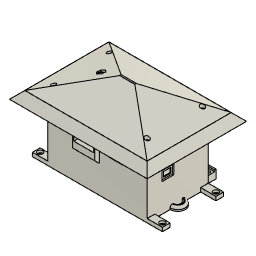
Smart Garden Enclosure v9 (Autodesk Fusion 360 design; units mm, degrees)
Autodesk Fusion 360 part; units mm, degrees
note: some values were not read from the file. Set by a fixed rule: which face or edge a step refers to.
(part 1 of 2)
sketch "Sketch1" plane through (0, 0, 0) normal (0, 0, 1) x (1, 0, 0)
  line L0 (0, 0) -> (130, 0)
  line L1 (130, 0) -> (130, 80)
  line L2 (130, 80) -> (0, 80)
  line L3 (0, 80) -> (0, 0)
  dimension "d1" = 130
  dimension "d2" = 80
  constraint horizontal L0
  constraint vertical L1
  constraint horizontal L2
  constraint vertical L3
  constraint coincident L0.start L3.end
  measures "d1" distance of L0.start L0.end
  measures "d2" distance of L0.start L2.end
extrude "Extrude1" add sketch "Sketch1" along normal blind 60 makes body 1
shell "Shell1" thickness 2 removed faces 1 at (43.3333, 26.6667, 60) on bodies 1
extrude "Extrude2" add 1 faces at (44, 52.6667, 2) along direction (0, 0, 1) blind 8 on bodies 1 bodies 1
sketch "Sketch2" plane through (0, 0, 0) normal (0, -1, 0) x (1, 0, 0)
  line L0 (0, 0) -> (130, 0)
  line L1 (130, 0) -> (130, 60)
  line L2 (130, 60) -> (0, 60)
  line L3 (0, 60) -> (0, 0)
  line L4 (2, 10) -> (128, 10)
  line L5 (128, 10) -> (2, 10)
  line L6 (4.76, 10) -> (125.26, 10)
  line L7 (4.76, 10) -> (4.76, 13.5)
  line L8 (4.76, 13.5) -> (125.26, 13.5)
  line L9 (125.26, 13.5) -> (125.26, 10)
  line L10 (16.01, 13.5) -> (33.01, 13.5)
  line L11 (33.01, 13.5) -> (33.01, 25)
  line L12 (33.01, 25) -> (16.01, 25)
  line L13 (16.01, 25) -> (16.01, 13.5)
  line L14 (43.01, 13.5) -> (60.01, 13.5)
  line L15 (60.01, 13.5) -> (60.01, 25)
  line L16 (60.01, 25) -> (43.01, 25)
  line L17 (43.01, 25) -> (43.01, 13.5)
  line L18 (70.01, 13.5) -> (87.01, 13.5)
  line L19 (87.01, 13.5) -> (87.01, 25)
  line L20 (87.01, 25) -> (70.01, 25)
  line L21 (70.01, 25) -> (70.01, 13.5)
  line L22 (97.01, 13.5) -> (114.01, 13.5)
  line L23 (114.01, 13.5) -> (114.01, 25)
  line L24 (114.01, 25) -> (97.01, 25)
  line L25 (97.01, 25) -> (97.01, 13.5)
  dimension "d27" = 120.5
  dimension "d29" = 3.5
  dimension "d30" = 17
  dimension "d31" = 11.5
  dimension "d32" = 17
  dimension "d33" = 11.5
  dimension "d35" = 17
  dimension "d36" = 11.5
  dimension "d37" = 17
  dimension "d38" = 11.5
  dimension "d42" = 11.25
  dimension "d43" = 11.25
  dimension "d44" = 10
  dimension "d45" = 10
  constraint coincident L4 L6.start
  constraint parallel L5 L6
  constraint perpendicular L5 L7
  constraint perpendicular L7 L8
  constraint perpendicular L8 L9
  constraint horizontal L10
  constraint vertical L11
  constraint horizontal L12
  constraint vertical L13
  constraint coincident L8 L10.start
  constraint horizontal L14
  constraint vertical L15
  constraint horizontal L16
  constraint vertical L17
  constraint coincident L8 L14.start
  constraint horizontal L18
  constraint vertical L19
  constraint horizontal L20
  constraint vertical L21
  constraint coincident L8 L18.start
  constraint horizontal L22
  constraint vertical L23
  constraint horizontal L24
  constraint vertical L25
  constraint coincident L8 L22.start
  measures "d27" distance of L6.start L6.end
  measures "d29" distance of L6.start L7.end
  measures "d30" distance of L10.start L10.end
  measures "d31" distance of L10.start L12.end
  measures "d32" distance of L14.start L14.end
  measures "d33" distance of L14.start L16.end
  measures "d35" distance of L18.start L18.end
  measures "d36" distance of L18.start L20.end
  measures "d37" distance of L22.start L22.end
  measures "d38" distance of L22.start L24.end
  measures "d42" distance of L9 L23
  measures "d43" distance of L7 L13
  measures "d44" distance of L11 L17
  measures "d45" distance of L15 L21
extrude "Extrude4" cut sketch "Sketch2" against normal blind 95 contours L4 L5 L6 L7 L8 L9 L10 L14 L18 L22 | L8 L10 L11 L12 L13 | L8 L22 L23 L24 L25 | L8 L14 L15 L16 L17 | L8 L18 L19 L20 L21 bodies 1
sketch "Sketch3" plane through (0, 0, 0) normal (0, -1, 0) x (1, 0, 0)
  line L0 (97.01, 25) -> (114.01, 25)
  line L1 (114.01, 25) -> (114.01, 13.5)
  line L2 (114.01, 13.5) -> (125.26, 13.5)
  line L3 (125.26, 13.5) -> (125.26, 10)
  line L4 (125.26, 10) -> (4.76, 10)
  line L5 (4.76, 10) -> (4.76, 13.5)
  line L6 (4.76, 13.5) -> (16.01, 13.5)
  line L7 (16.01, 13.5) -> (16.01, 25)
  line L8 (16.01, 25) -> (33.01, 25)
  line L9 (33.01, 25) -> (33.01, 13.5)
  line L10 (33.01, 13.5) -> (43.01, 13.5)
  line L11 (43.01, 13.5) -> (43.01, 25)
  line L12 (43.01, 25) -> (60.01, 25)
  line L13 (60.01, 25) -> (60.01, 13.5)
  line L14 (60.01, 13.5) -> (70.01, 13.5)
  line L15 (70.01, 13.5) -> (70.01, 25)
  line L16 (70.01, 25) -> (87.01, 25)
  line L17 (87.01, 25) -> (87.01, 13.5)
  line L18 (87.01, 13.5) -> (97.01, 13.5)
  line L19 (97.01, 13.5) -> (97.01, 25)
  line L20 (0, 0) -> (130, 0)
  line L21 (130, 0) -> (130, 60)
  line L22 (130, 60) -> (0, 60)
  line L23 (0, 60) -> (0, 0)
  line L24 (4.76, 10) -> (125.26, 10)
  line L25 (125.26, 10) -> (125.26, 0)
  line L26 (4.76, 10) -> (4.76, 0)
  constraint coincident L4.end L5.start
  constraint coincident L3.end L4.start
  constraint coincident L20 L25.end
  constraint perpendicular L20 L25
  constraint coincident L20 L26.end
  constraint perpendicular L20 L26
extrude "Extrude5" add sketch "Sketch3" against normal blind 93 contours L4 L20 L24 L25 L26 bodies 1
sketch "Sketch4" plane through (0, 0, 10) normal (0, 0, 1) x (-1, 0, 0)
  line L0 (-125.26, -2) -> (-128, -2)
  line L1 (-128, -2) -> (-128, -78)
  line L2 (-128, -78) -> (-125.26, -78)
  line L3 (-2, -78) -> (-2, -2)
  line L4 (-2, -2) -> (-4.76, -2)
  line L5 (-4.76, -2) -> (-4.76, 0)
  line L6 (-4.76, -93) -> (-4.76, -80)
  line L7 (-125.26, -80) -> (-125.26, -93)
  line L8 (-125.26, 0) -> (-125.26, -2)
  circle A0 centre (-9.51, 7.0656) radius 2
  circle A1 centre (-120.51, 6.9823) radius 2
  line L9 (-125.26, -93) -> (-4.76, -93)
  line L10 (-4.76, -78) -> (-2, -78)
  line L11 (-4.76, 0) -> (-125.26, 0)
  line L12 (-125.26, -78) -> (-125.26, -80)
  line L13 (-4.76, -80) -> (-4.76, -78)
  dimension "d51" = 4
  dimension "d52" = 4
  dimension "d53" = 111
  dimension "d54" = 4.75
  measures "d51" diameter of A0
  measures "d52" diameter of A1
  measures "d53" horizontal distance of A0.centre A1.centre
  measures "d54" distance of L6 A0.centre
extrude "Extrude6" cut sketch "Sketch4" against normal blind 6 contours A0 | A1 bodies 1
sketch "Sketch5" plane through (0, 0, 10) normal (0, 0, 1) x (-1, 0, 0)
  line L0 (-125.26, -2) -> (-128, -2)
  line L1 (-128, -2) -> (-128, -78)
  line L2 (-128, -78) -> (-125.26, -78)
  line L3 (-2, -78) -> (-2, -2)
  line L4 (-2, -2) -> (-4.76, -2)
  line L5 (-4.76, -2) -> (-4.76, 0)
  line L6 (-4.76, -93) -> (-4.76, -80)
  line L7 (-125.26, -80) -> (-125.26, -93)
  line L8 (-125.26, 0) -> (-125.26, -2)
  line L9 (-9.51, 7.0656) -> (-9.51, -78)
  line L10 (-120.51, 6.9823) -> (-120.51, -78)
  circle A0 centre (-9.51, -44.9344) radius 2
  circle A1 centre (-120.51, -45.0177) radius 2
  line L11 (-125.26, -93) -> (-4.76, -93)
  line L12 (-4.76, -78) -> (-2, -78)
  line L13 (-4.76, 0) -> (-125.26, 0)
  line L14 (-125.26, -78) -> (-125.26, -80)
  line L15 (-4.76, -80) -> (-4.76, -78)
  dimension "d57" = 4
  dimension "d58" = 4
  dimension "d59" = 52
  dimension "d60" = 52
  constraint coincident L2 L9.end
  constraint perpendicular L2 L9
  constraint coincident L2 L10.end
  constraint perpendicular L2 L10
  constraint coincident L9 A0.centre
  constraint coincident L10 A1.centre
  measures "d57" diameter of A0
  measures "d58" diameter of A1
  measures "d59" distance of L9.start A0.centre
  measures "d60" distance of L10.start A1.centre
extrude "Extrude7" cut sketch "Sketch5" against normal blind 5 contours L9 A0 | L9 A0 | L10 A1 | L10 A1 bodies 1
ref_plane "WorkPlane1" through (65, 46.5, 28) normal (0, 0, 1) x (1, 0, 0)
sketch "Sketch6" plane through (65, 32.5, 28) normal (0, 0, 1) x (1, 0, 0)
  line L0 (-63, 45.5) -> (63, 45.5)
  line L1 (63, 45.5) -> (63, -30.5)
  line L2 (63, -30.5) -> (-63, -30.5)
  line L3 (-63, -30.5) -> (-63, 45.5)
  line L4 (-65, 47.5) -> (-65, -32.5)
  line L5 (-65, -32.5) -> (65, -32.5)
  line L6 (65, -32.5) -> (65, 47.5)
  line L7 (65, 47.5) -> (-65, 47.5)
  line L8 (-63, -30.5) -> (-63, 45.5)
  line L9 (-63, -30.5) -> (-53, -30.5)
  line L10 (-53, -30.5) -> (-53, 45.5)
  line L11 (-53, 45.5) -> (-63, 45.5)
  line L12 (-53, -30.5) -> (-53, -18.5)
  line L13 (-53, -18.5) -> (-63, -18.5)
  line L14 (-53, 45.5) -> (-53, 30)
  line L15 (-53, 45.5) -> (-53, 33.5)
  line L16 (-53, 33.5) -> (-63, 33.5)
  line L17 (63, -30.5) -> (53, -30.5)
  line L18 (53, -30.5) -> (53, -18.5)
  line L19 (53, -18.5) -> (63, -18.5)
  line L20 (53, 45.5) -> (63, 45.5)
  line L21 (53, 45.5) -> (53, 33.5)
  line L22 (53, 33.5) -> (63, 33.5)
  line L23 (-53, -18.5) -> (-40, -18.5)
  line L24 (-40, -18.5) -> (-40, -30.5)
  line L25 (53, -18.5) -> (40, -18.5)
  line L26 (40, -18.5) -> (40, -30.5)
  line L27 (-53, 33.5) -> (-40, 33.5)
  line L28 (-40, 33.5) -> (-40, 45.5)
  line L29 (53, 33.5) -> (40, 33.5)
  line L30 (40, 33.5) -> (40, 45.5)
  dimension "d64" = 10
  dimension "d67" = 12
  dimension "d68" = 10
  dimension "d69" = 12
  dimension "d283" = 12
  dimension "d284" = 12
  constraint coincident L2.end L3.start
  constraint coincident L0.start L3.end
  constraint coincident L2 L9.end
  constraint perpendicular L3 L9
  constraint coincident L0 L10.end
  constraint perpendicular L0 L10
  constraint coincident L10 L12.end
  constraint perpendicular L9 L12
  constraint coincident L8 L13.end
  constraint perpendicular L8 L13
  constraint coincident L10 L14.end
  constraint perpendicular L11 L14
  constraint perpendicular L11 L15
  constraint coincident L8 L16.end
  constraint perpendicular L8 L16
  constraint coincident L1.end L2.start
  constraint coincident L2 L17.end
  constraint perpendicular L2 L18
  constraint coincident L1 L19.end
  constraint perpendicular L1 L19
  constraint coincident L0 L20.start
  constraint coincident L0.end L1.start
  constraint perpendicular L1 L20
  constraint perpendicular L20 L21
  constraint coincident L1 L22.end
  constraint perpendicular L1 L22
  constraint perpendicular L10 L23
  constraint coincident L2 L24.end
  constraint perpendicular L2 L24
  constraint perpendicular L18 L25
  constraint coincident L2 L26.end
  constraint perpendicular L2 L26
  constraint perpendicular L14 L27
  constraint coincident L0 L28.end
  constraint perpendicular L0 L28
  constraint perpendicular L21 L29
  constraint coincident L0 L30.end
  constraint perpendicular L0 L30
  measures "d64" distance of L8 L10
  measures "d67" distance of L10.end L15.end
  measures "d68" distance of L1.end L17.end
  measures "d69" distance of L20.start L21.end
  measures "d283" distance of L17 L19
  measures "d284" distance of L9 L13
extrude "Extrude8" add sketch "Sketch6" along normal blind 5 and the other way blind 7 contours L0 L3 L8 L10 L11 L14 L15 L16 | L2 L3 L8 L9 L10 L12 L13 | L0 L1 L20 L21 L22 | L1 L2 L17 L18 L19 bodies 1
sketch "Sketch7" plane through (0, 0, 33) normal (0, 0, 1) x (-1, 0, 0)
  line L0 (-2, -2) -> (-12, -2)
  line L1 (-12, -14) -> (-2, -14)
  line L2 (-2, -14) -> (-2, -2)
  line L3 (-12, -78) -> (-2, -78)
  line L4 (-2, -78) -> (-2, -66)
  line L5 (-2, -66) -> (-12, -66)
  line L6 (-118, -66) -> (-128, -66)
  line L7 (-128, -66) -> (-128, -78)
  line L8 (-128, -78) -> (-118, -78)
  line L9 (-118, -2) -> (-128, -2)
  line L10 (-128, -2) -> (-128, -14)
  line L11 (-128, -14) -> (-118, -14)
  line L12 (-2, -2) -> (-128, -2)
  line L13 (-128, -2) -> (-128, -78)
  line L14 (-128, -78) -> (-2, -78)
  line L15 (-2, -78) -> (-2, -2)
  line L16 (-3, -77) -> (-3, -3)
  line L17 (-3, -3) -> (-127, -3)
  line L18 (-127, -3) -> (-127, -77)
  line L19 (-127, -77) -> (-3, -77)
  line L20 (-12, -2) -> (-12, -14)
  line L21 (-12, -66) -> (-12, -78)
  line L22 (-118, -78) -> (-118, -66)
  line L23 (-118, -14) -> (-118, -2)
  dimension "d71" = -1
  constraint horizontal L12
  constraint vertical L13
  constraint horizontal L14
  constraint vertical L15
  constraint coincident L7.end L8.start
  constraint coincident L0.start L2.end
extrude "Extrude9" add sketch "Sketch7" along normal blind 7 separate body contours L1 L5 L6 L11 L16 L17 L18 L19 L20 L21 L22 L23 | L1 L16 L17 L20 | L11 L17 L18 L23 | L5 L16 L19 L21 | L6 L18 L19 L22 makes body 2
sketch "Sketch8" plane through (0, 0, 40) normal (0, 0, 1) x (-1, 0, 0)
  line L0 (-127, -77) -> (-3, -77)
  line L1 (-3, -77) -> (-3, -3)
  line L2 (-3, -3) -> (-127, -3)
  line L3 (-127, -3) -> (-127, -77)
  line L4 (-12, -78) -> (-2, -78)
  line L5 (-2, -78) -> (-2, -66)
  line L6 (-2, -66) -> (-12, -66)
  line L7 (-2, -2) -> (-12, -2)
  line L8 (-12, -14) -> (-2, -14)
  line L9 (-2, -14) -> (-2, -2)
  line L10 (-118, -66) -> (-128, -66)
  line L11 (-128, -66) -> (-128, -78)
  line L12 (-128, -78) -> (-118, -78)
  line L13 (-118, -2) -> (-128, -2)
  line L14 (-128, -2) -> (-128, -14)
  line L15 (-128, -14) -> (-118, -14)
  circle A0 centre (-7, -71.7119) radius 1.5
  circle A1 centre (-6.9931, -7.787) radius 1.5
  circle A2 centre (-123.226, -7.2087) radius 1.5
  line L16 (-12, -66) -> (-12, -78)
  line L17 (-12, -2) -> (-12, -14)
  line L18 (-118, -78) -> (-118, -66)
  line L19 (-118, -14) -> (-118, -2)
  dimension "d74" = 3
  dimension "d75" = 3
  dimension "d77" = 3
  measures "d74" diameter of A0
  measures "d75" diameter of A1
  measures "d77" diameter of A2
sketch "Sketch9" plane through (0, 80, 0) normal (0, 1, 0) x (-1, 0, 0)
  line L0 (-4.76, 0) -> (0, 0)
  line L1 (0, 0) -> (0, 60)
  line L2 (0, 60) -> (-130, 60)
  line L3 (-130, 60) -> (-130, 0)
  line L4 (-127, 40) -> (-3, 40)
  line L5 (-3, 40) -> (-127, 40)
  line L6 (-114.01, 25) -> (-97.01, 25)
  line L7 (-97.01, 25) -> (-97.01, 13.5)
  line L8 (-97.01, 13.5) -> (-87.01, 13.5)
  line L9 (-87.01, 13.5) -> (-87.01, 25)
  line L10 (-87.01, 25) -> (-70.01, 25)
  line L11 (-70.01, 25) -> (-70.01, 13.5)
  line L12 (-70.01, 13.5) -> (-60.01, 13.5)
  line L13 (-60.01, 13.5) -> (-60.01, 25)
  line L14 (-60.01, 25) -> (-43.01, 25)
  line L15 (-43.01, 25) -> (-43.01, 13.5)
  line L16 (-43.01, 13.5) -> (-33.01, 13.5)
  line L17 (-33.01, 13.5) -> (-33.01, 25)
  line L18 (-33.01, 25) -> (-16.01, 25)
  line L19 (-16.01, 25) -> (-16.01, 13.5)
  line L20 (-16.01, 13.5) -> (-4.76, 13.5)
  line L21 (-4.76, 13.5) -> (-4.76, 10)
  line L22 (-125.26, 10) -> (-125.26, 13.5)
  line L23 (-125.26, 13.5) -> (-114.01, 13.5)
  line L24 (-114.01, 13.5) -> (-114.01, 25)
  line L25 (-4.76, 10) -> (-4.76, 0)
  line L26 (-130, 0) -> (-125.26, 0)
  line L27 (-125.26, 0) -> (-125.26, 10)
sketch "Sketch10" plane through (0, 0, 40) normal (0, 0, 1) x (-1, 0, 0)
  line L0 (-127, -77) -> (-3, -77)
  line L1 (-3, -77) -> (-3, -3)
  line L2 (-3, -3) -> (-127, -3)
  line L3 (-127, -3) -> (-127, -77)
  circle A0 centre (-7, -71.7119) radius 3.5
  circle A1 centre (-6.9931, -7.787) radius 3.5
  circle A2 centre (-123.226, -7.2087) radius 3.5
  dimension "d80" = 7
  dimension "d81" = 7
  dimension "d83" = 7
  measures "d80" diameter of A0
  measures "d81" diameter of A1
  measures "d83" diameter of A2
sketch "Sketch14" plane through (0, 0, 40) normal (0, 0, 1) x (-1, 0, 0)
  line L0 (-127, -77) -> (-3, -77)
  line L1 (-3, -77) -> (-3, -3)
  line L2 (-3, -3) -> (-127, -3)
  line L3 (-127, -3) -> (-127, -77)
  line L4 (-127, -77) -> (-30, -77)
  line L5 (-30, -77) -> (-30, -13)
  line L6 (-30, -13) -> (-127, -13)
  line L7 (-127, -13) -> (-127, -77)
  dimension "d101" = 97
  dimension "d102" = 64
  constraint horizontal L4
  constraint vertical L5
  constraint horizontal L6
  constraint vertical L7
  constraint coincident L0.start L3.end
  measures "d101" distance of L0.start L4.end
  measures "d102" distance of L0.start L6.end
extrude "Extrude15" cut sketch "Sketch14" against normal blind 2 contours L0 L3 L4 L5 L6 L7 bodies 2
sketch "Sketch15" plane through (128, 0, 0) normal (-1, 0, 0) x (0, -1, 0)
  line L0 (-78, 33) -> (-66, 33)
  line L1 (-66, 33) -> (-66, 21)
  line L2 (-78, 21) -> (-78, 10)
  line L3 (-78, 10) -> (-2, 10)
  line L4 (-2, 10) -> (-2, 21)
  line L5 (-14, 21) -> (-14, 33)
  line L6 (-14, 33) -> (-2, 33)
  line L7 (-2, 33) -> (-2, 60)
  line L8 (-2, 60) -> (-78, 60)
  line L9 (-78, 60) -> (-78, 33)
  line L10 (-32, 40) -> (-22.5, 40)
  line L11 (-22.5, 40) -> (-22.5, 46.5)
  line L12 (-22.5, 46.5) -> (-32, 46.5)
  line L13 (-32, 46.5) -> (-32, 40)
  line L14 (-66, 21) -> (-78, 21)
  line L15 (-2, 21) -> (-14, 21)
  point P0 (-77, 38)
  point P1 (-13, 38)
  dimension "d105" = 9.5
  dimension "d106" = 6.5
  constraint horizontal L10
  constraint vertical L11
  constraint horizontal L12
  constraint vertical L13
  measures "d105" distance of L10.start L10.end
  measures "d106" distance of L10.start L12.end
extrude "Extrude16" cut sketch "Sketch15" against normal blind 2 contours L10 L11 L12 L13 bodies 1
sketch "Sketch16" plane through (130, 0, 0) normal (1, 0, 0) x (0, 1, 0)
  line L0 (32, 40) -> (22.5, 40)
  line L1 (22.5, 40) -> (22.5, 46.5)
  line L2 (22.5, 46.5) -> (32, 46.5)
  line L3 (32, 46.5) -> (32, 40)
  line L4 (0, 0) -> (80, 0)
  line L5 (80, 0) -> (80, 60)
  line L6 (80, 60) -> (0, 60)
  line L7 (0, 60) -> (0, 0)
  line L8 (34, 38) -> (20.5, 38)
  line L9 (20.5, 38) -> (20.5, 48.5)
  line L10 (20.5, 48.5) -> (34, 48.5)
  line L11 (34, 48.5) -> (34, 38)
  dimension "d110" = -2
extrude "Extrude17" cut sketch "Sketch16" against normal blind 1 contours L8 L9 L10 L11 bodies 1
chamfer "Chamfer4" distance 1 angle 45 4 edges at (130, 27.25, 48.5) (130, 34, 43.25) (130, 20.5, 43.25) (130, 27.25, 38) on bodies 1
sketch "Sketch17" plane through (0, 80, 0) normal (0, 1, 0) x (-1, 0, 0)
  line L0 (-117, 41) -> (-101.5, 41)
  line L1 (-101.5, 41) -> (-101.5, 49)
  line L2 (-101.5, 49) -> (-117, 49)
  line L3 (-117, 49) -> (-117, 41)
  line L4 (-96.5, 41) -> (-81, 41)
  line L5 (-81, 41) -> (-81, 49)
  line L6 (-81, 49) -> (-96.5, 49)
  line L7 (-96.5, 49) -> (-96.5, 41)
  line L8 (-76, 41) -> (-60.5, 41)
  line L9 (-60.5, 41) -> (-60.5, 49)
  line L10 (-60.5, 49) -> (-76, 49)
  line L11 (-76, 49) -> (-76, 41)
  line L12 (-55.5, 41) -> (-40, 41)
  line L13 (-40, 41) -> (-40, 49)
  line L14 (-40, 49) -> (-55.5, 49)
  line L15 (-55.5, 49) -> (-55.5, 41)
  line L16 (-127, 38) -> (-30, 38)
  line L17 (-30, 38) -> (-127, 38)
  point P0 (-127, 40)
  dimension "d114" = 15.5
  dimension "d115" = 8
  dimension "d116" = 10
  dimension "d117" = 15.5
  dimension "d118" = 8
  dimension "d119" = 15.5
  dimension "d120" = 8
  dimension "d121" = 15.5
  dimension "d122" = 8
  dimension "d123" = 5
  dimension "d124" = 5
  dimension "d125" = 5
  dimension "d126" = 3
  dimension "d127" = 3
  dimension "d128" = 3
  dimension "d129" = 3
  constraint horizontal L0
  constraint vertical L1
  constraint horizontal L2
  constraint vertical L3
  constraint horizontal L4
  constraint vertical L5
  constraint horizontal L6
  constraint vertical L7
  constraint horizontal L8
  constraint vertical L9
  constraint horizontal L10
  constraint vertical L11
  constraint horizontal L12
  constraint vertical L13
  constraint horizontal L14
  constraint vertical L15
  measures "d114" distance of L0.start L0.end
  measures "d115" distance of L0.start L2.end
  measures "d116" distance of L3 P0
  measures "d117" distance of L4.start L4.end
  measures "d118" distance of L4.start L6.end
  measures "d119" distance of L8.start L8.end
  measures "d120" distance of L8.start L10.end
  measures "d121" distance of L12.start L12.end
  measures "d122" distance of L12.start L14.end
  measures "d123" distance of L1 L7
  measures "d124" distance of L5 L11
  measures "d125" distance of L9 L15
  measures "d126" distance of L0 L17
  measures "d127" distance of L4 L16
  measures "d128" distance of L8 L17
  measures "d129" distance of L12 L16
extrude "Extrude18" cut sketch "Sketch17" against normal blind 2 bodies 1
chamfer "Chamfer5" distance 1 angle 45 12 edges at (24.51, 0, 25) (16.01, 0, 19.25) (33.01, 0, 19.25) (51.51, 0, 25) (60.01, 0, 19.25) (78.51, 0, 25) (87.01, 0, 19.25) (105.51, 0, 25) (114.01, 0, 19.25) (43.01, 0, 19.25) (70.01, 0, 19.25) (97.01, 0, 19.25) on bodies 1
chamfer "Chamfer6" distance 1 angle 45 5 edges at (9.885, 0, 13.5) (38.01, 0, 13.5) (65.01, 0, 13.5) (92.01, 0, 13.5) (120.135, 0, 13.5) on bodies 1
chamfer "Chamfer7" distance 1 angle 45 2 edges at (4.76, 0, 12.25) (125.26, 0, 12.25) on bodies 1
sketch "Sketch18" plane through (0, 80, 0) normal (0, 1, 0) x (-1, 0, 0)
  line L0 (-4.76, 0) -> (0, 0)
  line L1 (0, 0) -> (0, 60)
  line L2 (0, 60) -> (-130, 60)
  line L3 (-130, 60) -> (-130, 0)
  line L4 (-130, 50.5987) -> (-30, 50.5987)
  line L5 (-88.75, 50) -> (-88.75, 60)
  line L6 (-68.25, 50) -> (-68.25, 60)
  line L7 (-47.75, 50) -> (-47.75, 60)
  line L8 (-109.25, 50) -> (-109.25, 60)
  line L9 (-109.25, 55) -> (-47.75, 55)
  line L10 (-103.75, 58.5) -> (-114.75, 58.5)
  line L11 (-114.75, 58.5) -> (-114.75, 51.5)
  line L12 (-114.75, 51.5) -> (-103.75, 51.5)
  line L13 (-103.75, 51.5) -> (-103.75, 58.5)
  line L14 (-103.75, 58.5) -> (-114.75, 51.5) construction
  line L15 (-114.75, 58.5) -> (-103.75, 51.5) construction
  line L16 (-83.25, 58.5) -> (-94.25, 58.5)
  line L17 (-94.25, 58.5) -> (-94.25, 51.5)
  line L18 (-94.25, 51.5) -> (-83.25, 51.5)
  line L19 (-83.25, 51.5) -> (-83.25, 58.5)
  line L20 (-83.25, 58.5) -> (-94.25, 51.5) construction
  line L21 (-94.25, 58.5) -> (-83.25, 51.5) construction
  line L22 (-62.75, 58.5) -> (-73.75, 58.5)
  line L23 (-73.75, 58.5) -> (-73.75, 51.5)
  line L24 (-73.75, 51.5) -> (-62.75, 51.5)
  line L25 (-62.75, 51.5) -> (-62.75, 58.5)
  line L26 (-62.75, 58.5) -> (-73.75, 51.5) construction
  line L27 (-73.75, 58.5) -> (-62.75, 51.5) construction
  line L28 (-42.25, 58.5) -> (-53.25, 58.5)
  line L29 (-53.25, 58.5) -> (-53.25, 51.5)
  line L30 (-53.25, 51.5) -> (-42.25, 51.5)
  line L31 (-42.25, 51.5) -> (-42.25, 58.5)
  line L32 (-42.25, 58.5) -> (-53.25, 51.5) construction
  line L33 (-53.25, 58.5) -> (-42.25, 51.5) construction
  line L34 (-114.01, 25) -> (-97.01, 25)
  line L35 (-97.01, 25) -> (-97.01, 13.5)
  line L36 (-97.01, 13.5) -> (-87.01, 13.5)
  line L37 (-87.01, 13.5) -> (-87.01, 25)
  line L38 (-87.01, 25) -> (-70.01, 25)
  line L39 (-70.01, 25) -> (-70.01, 13.5)
  line L40 (-70.01, 13.5) -> (-60.01, 13.5)
  line L41 (-60.01, 13.5) -> (-60.01, 25)
  line L42 (-60.01, 25) -> (-43.01, 25)
  line L43 (-43.01, 25) -> (-43.01, 13.5)
  line L44 (-43.01, 13.5) -> (-33.01, 13.5)
  line L45 (-33.01, 13.5) -> (-33.01, 25)
  line L46 (-33.01, 25) -> (-16.01, 25)
  line L47 (-16.01, 25) -> (-16.01, 13.5)
  line L48 (-16.01, 13.5) -> (-4.76, 13.5)
  line L49 (-4.76, 13.5) -> (-4.76, 10)
  line L50 (-125.26, 10) -> (-125.26, 13.5)
  line L51 (-125.26, 13.5) -> (-114.01, 13.5)
  line L52 (-114.01, 13.5) -> (-114.01, 25)
  line L53 (-4.76, 10) -> (-4.76, 0)
  line L54 (-130, 0) -> (-125.26, 0)
  line L55 (-125.26, 0) -> (-125.26, 10)
  line L56 (-60.5, 41) -> (-76, 41)
  line L57 (-76, 41) -> (-76, 49)
  line L58 (-76, 49) -> (-60.5, 49)
  line L59 (-60.5, 49) -> (-60.5, 41)
  line L60 (-81, 41) -> (-96.5, 41)
  line L61 (-96.5, 41) -> (-96.5, 49)
  line L62 (-96.5, 49) -> (-81, 49)
  line L63 (-81, 49) -> (-81, 41)
  line L64 (-101.5, 41) -> (-117, 41)
  line L65 (-117, 41) -> (-117, 49)
  line L66 (-117, 49) -> (-101.5, 49)
  line L67 (-101.5, 49) -> (-101.5, 41)
  line L68 (-40, 41) -> (-55.5, 41)
  line L69 (-55.5, 41) -> (-55.5, 49)
  line L70 (-55.5, 49) -> (-40, 49)
  line L71 (-40, 49) -> (-40, 41)
  point P0 (-109.25, 55)
  point P1 (-88.75, 55)
  point P2 (-68.25, 55)
  point P3 (-47.75, 55)
  dimension "d138" = 11
  dimension "d139" = 7
  dimension "d140" = 11
  dimension "d141" = 7
  dimension "d142" = 11
  dimension "d143" = 7
  dimension "d144" = 11
  dimension "d145" = 7
  constraint coincident L3 L4.start
  constraint coincident L2 L5.end
  constraint perpendicular L2 L5
  constraint coincident L2 L6.end
  constraint perpendicular L2 L6
  constraint coincident L2 L7.end
  constraint perpendicular L2 L7
  constraint coincident L2 L8.end
  constraint perpendicular L2 L8
  constraint midpoint L8 P0
  constraint midpoint L7 P3
  constraint horizontal L10
  constraint perpendicular L10 L11
  constraint parallel L10 L12
  constraint parallel L11 L13
  constraint coincident L14 P0
  constraint coincident L15 P0
  constraint coincident P0 L9.start
  constraint horizontal L16
  constraint perpendicular L16 L17
  constraint parallel L16 L18
  constraint parallel L17 L19
  constraint coincident L20 P1
  constraint coincident L21 P1
  constraint midpoint L5 P1
  constraint horizontal L22
  constraint perpendicular L22 L23
  constraint parallel L22 L24
  constraint parallel L23 L25
  constraint coincident L26 P2
  constraint coincident L27 P2
  constraint midpoint L6 P2
  constraint horizontal L28
  constraint perpendicular L28 L29
  constraint parallel L28 L30
  constraint parallel L29 L31
  constraint coincident L32 P3
  constraint coincident L33 P3
  constraint coincident P3 L9.end
  measures "d138" distance of L11.end L12.end
  measures "d139" distance of L10.end L11.end
  measures "d140" distance of L17.end L18.end
  measures "d141" distance of L16.end L17.end
  measures "d142" distance of L23.end L24.end
  measures "d143" distance of L22.end L23.end
  measures "d144" distance of L29.end L30.end
  measures "d145" distance of L28.end L29.end
extrude "Extrude19" cut sketch "Sketch18" against normal blind 2 contours L7 L28 L30 L31 | L7 L9 L28 L29 | L6 L9 L22 L25 | L6 L9 L22 L23 | L7 L9 L29 L30 | L5 L9 L16 L19 | L5 L9 L16 L17 | L6 L9 L24 L25 | L6 L9 L23 L24 | L8 L9 L10 L13 | L8 L10 L11 L12 | L5 L9 L18 L19 | L5 L9 L17 L18 | L8 L9 L12 L13 bodies 1
sketch "Sketch19" plane through (0, 0, 38) normal (0, 0, 1) x (-1, 0, 0)
  line L0 (-127, -13) -> (-127, -77)
  line L1 (-127, -77) -> (-30, -77)
  line L2 (-30, -77) -> (-30, -13)
  line L3 (-30, -13) -> (-127, -13)
  circle A0 centre (-123.2, -73.2) radius 1.6
  line L4 (-123.2, -73.2) -> (-30, -73.2)
  line L5 (-123.2, -73.2) -> (-123.2, -13)
  circle A1 centre (-33.8, -73.2) radius 1.6
  circle A2 centre (-123.2, -16.8) radius 1.6
  line L6 (-33.8, -73.2) -> (-33.8, -13)
  line L7 (-123.2, -16.8) -> (-30, -16.8)
  circle A3 centre (-33.8, -16.8) radius 1.6
  dimension "d148" = 3.2
  dimension "d149" = 3.8
  dimension "d150" = 3.8
  dimension "d151" = 3.2
  dimension "d152" = 3.2
  dimension "d153" = 3.8
  dimension "d154" = 3.2
  dimension "d155" = 3.8
  constraint coincident A0.centre L4.start
  constraint coincident L2 L4.end
  constraint perpendicular L2 L4
  constraint coincident L3 L5.end
  constraint perpendicular L3 L5
  constraint coincident L4 A1.centre
  constraint coincident L5 A2.centre
  constraint coincident A1.centre L6.start
  constraint coincident L3 L6.end
  constraint perpendicular L3 L6
  constraint coincident A2.centre L7.start
  constraint coincident L2 L7.end
  constraint perpendicular L2 L7
  constraint coincident L6 A3.centre
  constraint coincident L7 A3.centre
  measures "d148" diameter of A0
  measures "d149" distance of L1 A0.centre
  measures "d150" distance of L0 A0.centre
  measures "d151" diameter of A1
  measures "d152" diameter of A2
  measures "d153" distance of L2 A1.centre
  measures "d154" diameter of A3
  measures "d155" distance of L3 A2.centre
extrude "Extrude20" cut sketch "Sketch19" against normal blind 5 contours L5 A2 L7 | L5 A2 | L6 L7 A3 | L6 L7 A3 | L5 A2 L7 | L4 A1 | L4 A1 L6 | L6 L7 A3 | L6 L7 A3 | L4 A1 L6 bodies 2
sketch "Sketch20" plane through (0, 0, 60) normal (0, 0, 1) x (-1, 0, 0)
  line L0 (-2, -78) -> (-128, -78)
  line L1 (-128, -78) -> (-128, -2)
  line L2 (-128, -2) -> (-2, -2)
  line L3 (-2, -2) -> (-2, -78)
  line L4 (0, -80) -> (0, 0)
  line L5 (0, 0) -> (-130, 0)
  line L6 (-130, 0) -> (-130, -80)
  line L7 (-130, -80) -> (0, -80)
extrude "Extrude21" add sketch "Sketch20" along normal blind 25 bodies 1
sketch "Sketch21" plane through (0, 0, 85) normal (0, 0, 1) x (-1, 0, 0)
  line L0 (-128, -2) -> (-2, -2)
  line L1 (-2, -2) -> (-2, -78)
  line L2 (-2, -78) -> (-128, -78)
  line L3 (-128, -78) -> (-128, -2)
  line L4 (-130, -80) -> (0, -80)
  line L5 (0, -80) -> (0, 0)
  line L6 (0, 0) -> (-130, 0)
  line L7 (-130, 0) -> (-130, -80)
  line L8 (25, -105) -> (25, 25)
  line L9 (25, 25) -> (-155, 25)
  line L10 (-155, 25) -> (-155, -105)
  line L11 (-155, -105) -> (25, -105)
  dimension "d160" = 25
extrude "Extrude22" add sketch "Sketch21" along normal blind 0 and the other way blind 10 contours L4 L5 L6 L7 | L8 L9 L10 L11 bodies 1
ref_plane "WorkPlane2" through (65, 40, 110) normal (0, 0, 1) x (1, 0, 0)
sketch "Sketch22" plane through (0, 0, 85) normal (0, 0, 1) x (-1, 0, 0)
  line L0 (-128, -2) -> (-2, -2)
  line L1 (-2, -2) -> (-2, -78)
  line L2 (-2, -78) -> (-128, -78)
  line L3 (-128, -78) -> (-128, -2)
  line L4 (-145, -95) -> (15, -95)
  line L5 (15, -95) -> (15, 15)
  line L6 (15, 15) -> (-145, 15)
  line L7 (-145, 15) -> (-145, -95)
sketch "Sketch23" plane through (65, 40, 110) normal (0, 0, 1) x (1, 0, 0)
  line L0 (10, -1) -> (-10, -1)
  line L1 (-10, -1) -> (-10, 1)
  line L2 (-10, 1) -> (10, 1)
  line L3 (10, 1) -> (10, -1)
  line L4 (10, -1) -> (-10, 1) construction
  line L5 (-10, -1) -> (10, 1) construction
  dimension "d169" = 20
  dimension "d170" = 2
  constraint horizontal L0
  constraint perpendicular L0 L1
  constraint parallel L0 L2
  constraint parallel L1 L3
  constraint coincident L4 origin
  constraint coincident L5 origin
  measures "d169" distance of L1.end L2.end
  measures "d170" distance of L0.end L1.end
extrude "Extrude24" add sketch "Sketch23" against normal blind 0.1 separate body makes body 3
sketch "Sketch26" plane through (0, 2, 0) normal (0, 1, 0) x (-1, 0, 0)
  line L0 (-128, 85) -> (-128, 33)
  line L1 (-128, 33) -> (-118, 33)
  line L2 (-128, 21) -> (-128, 10)
  line L3 (-128, 10) -> (-125.26, 10)
  line L4 (-125.26, 10) -> (-125.26, 13.5)
  line L5 (-125.26, 13.5) -> (-114.01, 13.5)
  line L6 (-114.01, 13.5) -> (-114.01, 25)
  line L7 (-114.01, 25) -> (-97.01, 25)
  line L8 (-97.01, 25) -> (-97.01, 13.5)
  line L9 (-97.01, 13.5) -> (-87.01, 13.5)
  line L10 (-87.01, 13.5) -> (-87.01, 25)
  line L11 (-87.01, 25) -> (-70.01, 25)
  line L12 (-70.01, 25) -> (-70.01, 13.5)
  line L13 (-70.01, 13.5) -> (-60.01, 13.5)
  line L14 (-60.01, 13.5) -> (-60.01, 25)
  line L15 (-60.01, 25) -> (-43.01, 25)
  line L16 (-43.01, 25) -> (-43.01, 13.5)
  line L17 (-43.01, 13.5) -> (-33.01, 13.5)
  line L18 (-33.01, 13.5) -> (-33.01, 25)
  line L19 (-33.01, 25) -> (-16.01, 25)
  line L20 (-16.01, 25) -> (-16.01, 13.5)
  line L21 (-16.01, 13.5) -> (-4.76, 13.5)
  line L22 (-4.76, 13.5) -> (-4.76, 10)
  line L23 (-4.76, 10) -> (-2, 10)
  line L24 (-2, 10) -> (-2, 21)
  line L25 (-2, 33) -> (-2, 85)
  line L26 (-2, 85) -> (-128, 85)
  line L27 (-67.5, 38.1042) -> (-38.5, 38.1042)
  line L28 (-38.5, 38.1042) -> (-38.5, 70.1042)
  line L29 (-38.5, 70.1042) -> (-67.5, 70.1042)
  line L30 (-67.5, 70.1042) -> (-67.5, 38.1042)
  line L31 (-66, 50.6042) -> (-40, 50.6042)
  line L32 (-40, 50.6042) -> (-40, 65.6042)
  line L33 (-40, 65.6042) -> (-66, 65.6042)
  line L34 (-66, 65.6042) -> (-66, 50.6042)
  line L35 (-98.5, 51.5884) -> (-80, 51.5884)
  line L36 (-80, 51.5884) -> (-80, 70.0884)
  line L37 (-80, 70.0884) -> (-98.5, 70.0884)
  line L38 (-98.5, 70.0884) -> (-98.5, 51.5884)
  line L39 (-89.25, 70.0884) -> (-89.25, 51.5884)
  line L40 (-80, 60.8384) -> (-98.5, 60.8384)
  line L41 (-86.25, 57.8384) -> (-92.25, 57.8384)
  line L42 (-92.25, 57.8384) -> (-92.25, 63.8384)
  line L43 (-92.25, 63.8384) -> (-86.25, 63.8384)
  line L44 (-86.25, 63.8384) -> (-86.25, 57.8384)
  line L45 (-86.25, 57.8384) -> (-92.25, 63.8384) construction
  line L46 (-92.25, 57.8384) -> (-86.25, 63.8384) construction
  line L47 (-118, 33) -> (-118, 21)
  line L48 (-118, 21) -> (-128, 21)
  line L49 (-2, 21) -> (-12, 21)
  line L50 (-12, 21) -> (-12, 33)
  line L51 (-12, 33) -> (-2, 33)
  point P0 (-89.25, 60.8384)
  dimension "d182" = 29
  dimension "d183" = 32
  dimension "d184" = 26
  dimension "d185" = 15
  dimension "d186" = 1.5
  dimension "d187" = 4.5
  dimension "d188" = 18.5
  dimension "d189" = 18.5
  dimension "d190" = 6
  dimension "d191" = 6
  dimension "d294" = 60
  dimension "d295" = 36.5
  constraint horizontal L27
  constraint vertical L28
  constraint horizontal L29
  constraint vertical L30
  constraint horizontal L31
  constraint vertical L32
  constraint horizontal L33
  constraint vertical L34
  constraint horizontal L35
  constraint vertical L36
  constraint horizontal L37
  constraint vertical L38
  constraint midpoint L37 L39.start
  constraint midpoint L35 L39.end
  constraint midpoint L36 L40.start
  constraint midpoint L38 L40.end
  constraint horizontal L41
  constraint perpendicular L41 L42
  constraint parallel L41 L43
  constraint parallel L42 L44
  constraint coincident L45 P0
  constraint coincident L46 P0
  constraint midpoint L39 P0
  measures "d182" distance of L27.start L27.end
  measures "d183" distance of L27.start L29.end
  measures "d184" distance of L31.start L31.end
  measures "d185" distance of L31.start L33.end
  measures "d186" distance of L28 L32
  measures "d187" distance of L29 L33
  measures "d188" distance of L35.start L35.end
  measures "d189" distance of L35.start L37.end
  measures "d190" distance of L42.end L43.end
  measures "d191" distance of L41.end L42.end
  measures "d294" distance of L28 L38
  measures "d295" distance of L25 L28
extrude "Extrude25" cut sketch "Sketch26" against normal blind 1 contours L27 L28 L29 L30 | L31 L32 L33 L34 bodies 1
extrude "Extrude26" cut sketch "Sketch26" against normal blind 1 contours L35 L38 L39 L40 L41 L42 | L35 L36 L39 L40 L41 L44 | L37 L38 L39 L40 L42 L43 | L39 L40 L41 L42 | L39 L40 L41 L44 | L39 L40 L42 L43 | L36 L37 L39 L40 L43 L44 | L39 L40 L43 L44 bodies 1
sketch "Sketch27" plane through (0, 0, 0) normal (0, -1, 0) x (1, 0, 0)
  line L0 (130, 75) -> (0, 75)
  line L1 (0, 75) -> (0, 0)
  line L2 (0, 0) -> (130, 0)
  line L3 (126.26, 10) -> (3.76, 10)
  line L4 (3.76, 10) -> (3.76, 14.5)
  line L5 (3.76, 14.5) -> (15.01, 14.5)
  line L6 (15.01, 14.5) -> (15.01, 26)
  line L7 (15.01, 26) -> (34.01, 26)
  line L8 (34.01, 26) -> (34.01, 14.5)
  line L9 (34.01, 14.5) -> (42.01, 14.5)
  line L10 (42.01, 14.5) -> (42.01, 26)
  line L11 (42.01, 26) -> (61.01, 26)
  line L12 (61.01, 26) -> (61.01, 14.5)
  line L13 (61.01, 14.5) -> (69.01, 14.5)
  line L14 (69.01, 14.5) -> (69.01, 26)
  line L15 (69.01, 26) -> (88.01, 26)
  line L16 (88.01, 26) -> (88.01, 14.5)
  line L17 (88.01, 14.5) -> (96.01, 14.5)
  line L18 (96.01, 14.5) -> (96.01, 26)
  line L19 (96.01, 26) -> (115.01, 26)
  line L20 (115.01, 26) -> (115.01, 14.5)
  line L21 (115.01, 14.5) -> (126.26, 14.5)
  line L22 (126.26, 14.5) -> (126.26, 10)
  line L23 (130, 0) -> (130, 75)
  line L24 (38.5, 38.1042) -> (38.5, 70.1042)
  line L25 (67.5, 38.1042) -> (38.5, 38.1042)
  line L26 (67.5, 70.1042) -> (67.5, 38.1042)
  line L27 (38.5, 70.1042) -> (67.5, 70.1042)
  line L28 (80, 51.5884) -> (80, 70.0884)
  line L29 (80, 70.0884) -> (98.5, 70.0884)
  line L30 (98.5, 70.0884) -> (98.5, 51.5884)
  line L31 (98.5, 51.5884) -> (80, 51.5884)
  line L32 (40, 65.6042) -> (66, 65.6042)
  line L33 (40, 50.6042) -> (40, 65.6042)
  line L34 (66, 50.6042) -> (40, 50.6042)
  line L35 (66, 65.6042) -> (66, 50.6042)
  line L36 (86.25, 63.8384) -> (86.25, 57.8384)
  line L37 (92.25, 63.8384) -> (86.25, 63.8384)
  line L38 (92.25, 57.8384) -> (92.25, 63.8384)
  line L39 (86.25, 57.8384) -> (92.25, 57.8384)
  line L40 (38.5, 38.1042) -> (38.5, 36.1042)
  line L41 (38.5, 36.1042) -> (67.5, 36.1042)
  line L42 (67.5, 36.1042) -> (67.5, 70.1042)
  line L43 (67.5, 70.1042) -> (67.5, 72.1042)
  line L44 (67.5, 72.1042) -> (38.5, 72.1042)
  line L45 (38.5, 72.1042) -> (38.5, 70.1042)
  line L46 (80, 51.5884) -> (80, 49.5884)
  line L47 (80, 49.5884) -> (98.5, 49.5884)
  line L48 (98.5, 49.5884) -> (98.5, 70.0884)
  line L49 (98.5, 70.0884) -> (98.5, 72.0884)
  line L50 (98.5, 72.0884) -> (80, 72.0884)
  line L51 (80, 72.0884) -> (80, 70.0884)
  dimension "d196" = 2
  dimension "d197" = 2
  dimension "d205" = 2
  dimension "d206" = 2
  constraint coincident L24.start L25.end
  constraint perpendicular L25 L40
  constraint perpendicular L26 L41
  constraint coincident L26.start L27.end
  constraint perpendicular L27 L42
  constraint perpendicular L27 L43
  constraint perpendicular L24 L44
  constraint coincident L24.end L27.start
  constraint perpendicular L27 L45
  constraint coincident L28.start L31.end
  constraint perpendicular L31 L46
  constraint perpendicular L30 L47
  constraint coincident L29.end L30.start
  constraint perpendicular L29 L48
  constraint perpendicular L29 L49
  constraint perpendicular L28 L50
  constraint coincident L28.end L29.start
  constraint perpendicular L29 L51
  measures "d196" distance of L24.start L40.end
  measures "d197" distance of L26.start L43.end
  measures "d205" distance of L28.start L46.end
  measures "d206" distance of L29.end L49.end
extrude "Extrude30" add sketch "Sketch27" along normal blind 3 contours L28 L29 L30 L31 L48 | L31 L46 L47 L48 | L29 L49 L50 L51 | L36 L37 L38 L39 bodies 1
extrude "Extrude27" add sketch "Sketch27" along normal blind 6 contours L24 L25 L26 L27 L42 | L25 L40 L41 L42 | L27 L43 L44 L45 | L32 L33 L34 L35 bodies 1
chamfer "Chamfer10" distance 6 angle 45 2 edges at (53, -6, 72.1042) (53, -6, 36.1042) on bodies 1
extrude "Extrude28" cut sketch "Sketch26" against normal blind 2 contours L27 L28 L29 L30 bodies 1
extrude "Extrude29" cut sketch "Sketch26" against normal blind 11 contours L31 L32 L33 L34 bodies 1
chamfer "Chamfer11" distance 3 angle 45 4 edges at (89.25, -3, 72.0884) (89.25, -3, 49.5884) (80, -3, 60.8384) (98.5, -3, 60.8384) on bodies 1
extrude "Extrude31" cut sketch "Sketch26" against normal blind 2 contours L35 L38 L39 L40 L41 L42 | L35 L36 L39 L40 L41 L44 | L37 L38 L39 L40 L42 L43 | L36 L37 L39 L40 L43 L44 bodies 1
extrude "Extrude32" cut sketch "Sketch26" against normal blind 6 contours L39 L40 L41 L42 | L39 L40 L41 L44 | L39 L40 L42 L43 | L39 L40 L43 L44 bodies 1
sketch "Sketch28" plane through (0, 2, 0) normal (0, 1, 0) x (-1, 0, 0)
  line L0 (-80, 51.5884) -> (-98.5, 51.5884)
  line L1 (-98.5, 51.5884) -> (-98.5, 70.0884)
  line L2 (-98.5, 70.0884) -> (-80, 70.0884)
  line L3 (-80, 70.0884) -> (-80, 51.5884)
  line L4 (-67.5, 38.1042) -> (-67.5, 70.1042)
  line L5 (-67.5, 70.1042) -> (-38.5, 70.1042)
  line L6 (-38.5, 70.1042) -> (-38.5, 38.1042)
  line L7 (-128, 85) -> (-128, 33)
  line L8 (-128, 33) -> (-118, 33)
  line L9 (-128, 21) -> (-128, 10)
  line L10 (-128, 10) -> (-125.26, 10)
  line L11 (-125.26, 10) -> (-125.26, 13.5)
  line L12 (-125.26, 13.5) -> (-114.01, 13.5)
  line L13 (-114.01, 13.5) -> (-114.01, 25)
  line L14 (-114.01, 25) -> (-97.01, 25)
  line L15 (-97.01, 25) -> (-97.01, 13.5)
  line L16 (-97.01, 13.5) -> (-87.01, 13.5)
  line L17 (-87.01, 13.5) -> (-87.01, 25)
  line L18 (-87.01, 25) -> (-70.01, 25)
  line L19 (-70.01, 25) -> (-70.01, 13.5)
  line L20 (-70.01, 13.5) -> (-60.01, 13.5)
  line L21 (-60.01, 13.5) -> (-60.01, 25)
  line L22 (-60.01, 25) -> (-43.01, 25)
  line L23 (-33.01, 25) -> (-16.01, 25)
  line L24 (-16.01, 25) -> (-16.01, 13.5)
  line L25 (-16.01, 13.5) -> (-4.76, 13.5)
  line L26 (-4.76, 13.5) -> (-4.76, 10)
  line L27 (-4.76, 10) -> (-2, 10)
  line L28 (-2, 10) -> (-2, 21)
  line L29 (-2, 33) -> (-2, 85)
  line L30 (-2, 85) -> (-128, 85)
  line L31 (-65.3334, 49.6911) -> (-38.5, 49.6911)
  line L32 (-118, 33) -> (-118, 21)
  line L33 (-118, 21) -> (-128, 21)
  line L34 (-2, 21) -> (-12, 21)
  line L35 (-12, 21) -> (-12, 33)
  line L36 (-12, 33) -> (-2, 33)
  line L37 (-38.5, 38.1042) -> (-67.5, 38.1042)
  line L38 (-43.01, 25) -> (-43.01, 13.5)
  line L39 (-43.01, 13.5) -> (-33.01, 13.5)
  line L40 (-33.01, 13.5) -> (-33.01, 25)
  constraint coincident L6 L31.end
  constraint perpendicular L6 L31
sketch "Sketch29" plane through (0, 0, 0) normal (0, 1, 0) x (-1, 0, 0)
  line L0 (-92.25, 63.8384) -> (-86.25, 63.8384)
  line L1 (-86.25, 63.8384) -> (-86.25, 57.8384)
  line L2 (-86.25, 57.8384) -> (-92.25, 57.8384)
  line L3 (-92.25, 57.8384) -> (-92.25, 63.8384)
  line L4 (-98.5, 70.0884) -> (-98.5, 51.5884)
  line L5 (-98.5, 51.5884) -> (-80, 51.5884)
  line L6 (-80, 51.5884) -> (-80, 70.0884)
  line L7 (-80, 70.0884) -> (-98.5, 70.0884)
  circle A0 centre (-82, 53.5884) radius 1
  line L8 (-82, 53.5884) -> (-82, 70.0884)
  line L9 (-82, 53.5884) -> (-98.5, 53.5884)
  line L10 (-82, 68.0884) -> (-98.5, 68.0884)
  line L11 (-98.5, 70.0884) -> (-80, 70.0884)
  line L12 (-96.5, 70.0884) -> (-96.5, 53.5884)
  circle A1 centre (-96.5, 68.0884) radius 1
  circle A2 centre (-82, 68.0884) radius 1
  circle A3 centre (-96.5, 53.5884) radius 1
  dimension "d218" = 2
  dimension "d219" = 2
  dimension "d220" = 2
  dimension "d221" = 2
  dimension "d222" = 2
  dimension "d223" = 2
  dimension "d224" = 2
  dimension "d225" = 2
  constraint coincident A0.centre L8.start
  constraint coincident L7 L8.end
  constraint perpendicular L7 L8
  constraint coincident L4 L9.end
  constraint perpendicular L4 L9
  constraint coincident L8 L10.start
  constraint coincident L4 L10.end
  constraint perpendicular L4 L10
  constraint coincident L11 L12.start
  constraint coincident L9 L12.end
  constraint perpendicular L9 L12
  constraint coincident L12 A1.centre
  constraint coincident L10 A1.centre
  constraint coincident L10.start A2.centre
  constraint coincident L12.end A3.centre
  measures "d218" diameter of A0
  measures "d219" distance of L5 A0.centre
  measures "d220" distance of L6 A0.centre
  measures "d221" distance of L10 L11
  measures "d222" distance of L4 L12
  measures "d223" diameter of A1
  measures "d224" diameter of A2
  measures "d225" diameter of A3
sketch "Sketch30" plane through (0, -3, 0) normal (0, -1, 0) x (1, 0, 0)
  line L0 (92.25, 63.8384) -> (92.25, 57.8384)
  line L1 (92.25, 57.8384) -> (86.25, 57.8384)
  line L2 (86.25, 57.8384) -> (86.25, 63.8384)
  line L3 (86.25, 63.8384) -> (92.25, 63.8384)
  line L4 (83, 52.5884) -> (95.5, 52.5884)
  line L5 (95.5, 52.5884) -> (95.5, 69.0884)
  line L6 (95.5, 69.0884) -> (83, 69.0884)
  line L7 (83, 69.0884) -> (83, 52.5884)
  line L8 (98.5, 70.0884) -> (98.5, 72.0884)
  line L9 (98.5, 72.0884) -> (95.5, 69.0884)
  line L10 (95.5, 69.0884) -> (95.5, 52.5884)
  line L11 (95.5, 52.5884) -> (98.5, 49.5884)
  line L12 (98.5, 51.5884) -> (98.5, 70.0884)
  line L13 (83, 52.5884) -> (83, 69.0884)
  line L14 (83, 69.0884) -> (80, 72.0884)
  line L15 (80, 72.0884) -> (80, 70.0884)
  line L16 (80, 70.0884) -> (80, 51.5884)
  line L17 (80, 51.5884) -> (80, 49.5884)
  line L18 (80, 49.5884) -> (83, 52.5884)
  circle A0 centre (89.5, 44.333) radius 3
  circle A1 centre (89.5, 58.833) radius 3
  circle A2 centre (75, 58.833) radius 3
  circle A3 centre (75, 44.333) radius 3
  line L19 (98.5, 49.5884) -> (98.5, 51.5884)
  dimension "d228" = 6
  dimension "d231" = 6
  dimension "d232" = 6
  dimension "d233" = 6
  measures "d228" diameter of A0
  measures "d231" diameter of A1
  measures "d232" diameter of A2
  measures "d233" diameter of A3
sketch "Sketch31" plane through (0, -6, 0) normal (0, -1, 0) x (1, 0, 0)
  line L0 (66, 50.6042) -> (40, 50.6042)
  line L1 (40, 50.6042) -> (40, 65.6042)
  line L2 (40, 65.6042) -> (66, 65.6042)
  line L3 (66, 65.6042) -> (66, 50.6042)
  line L4 (38.5, 42.1042) -> (67.5, 42.1042)
  line L5 (67.5, 42.1042) -> (67.5, 66.1042)
  line L6 (67.5, 66.1042) -> (38.5, 66.1042)
  line L7 (38.5, 66.1042) -> (38.5, 42.1042)
  line L8 (67.5, 36.1042) -> (67.5, 42.1042)
  line L9 (67.5, 42.1042) -> (38.5, 42.1042)
  line L10 (38.5, 42.1042) -> (38.5, 36.1042)
  line L11 (38.5, 36.1042) -> (67.5, 36.1042)
chamfer "Chamfer13" distance 10 angle 45 4 edges at (65, -25, 85) (-25, 40, 85) (65, 105, 85) (155, 40, 85) on bodies 1
sketch "Sketch32" plane through (0, 0, 85) normal (0, 0, 1) x (-1, 0, 0)
  line L0 (-128, -2) -> (-2, -2)
  line L1 (-2, -2) -> (-2, -78)
  line L2 (-2, -78) -> (-128, -78)
  line L3 (-128, -78) -> (-128, -2)
  line L4 (-145, -95) -> (15, -95)
  line L5 (15, -95) -> (15, 15)
  line L6 (15, 15) -> (-145, 15)
  line L7 (-145, 15) -> (-145, -95)
extrude "Extrude38" add sketch "Sketch32" 1 faces at (44, 89.3347, 85) along normal blind 0.1 contours L0 L1 L2 L3 on bodies 1 bodies 1
loft "Loft2" add section 1 face at (91.6673, 58.334, 85.1) section 2 face at (61.6667, 39.6667, 109.9) on bodies 1 3 bodies 1 3
ref_plane "WorkPlane3" through (65, 40, 75) normal (0, 0, 1) x (1, 0, 0)
split "Split1" by plane through (65, 40, 75) normal (0, 0, 1) bodies 1 makes body 4 at (43.3333, 96.6667, 75)
move_body "Move3" bodies 4 to x (1, 0, 0) y (0, 1, 0) z (0, 0, 1) at (0, 0, 25)
sketch "Sketch33" plane through (0, 0, 100) normal (0, 0, -1) x (1, 0, 0)
  line L0 (2, -78) -> (2, -2)
  line L1 (2, -2) -> (128, -2)
  line L2 (128, -2) -> (128, -78)
  line L3 (128, -78) -> (2, -78)
  line L4 (-25, -105) -> (155, -105)
  line L5 (155, -105) -> (155, 25)
  line L6 (155, 25) -> (-25, 25)
  line L7 (-25, 25) -> (-25, -105)
  line L8 (2, -2) -> (2, -78)
  line L9 (2, -78) -> (128, -78)
  line L10 (128, -78) -> (128, -2)
  line L11 (128, -2) -> (2, -2)
  line L12 (1.4, -78.6) -> (128.6, -78.6)
  line L13 (128.6, -78.6) -> (128.6, -1.4)
  line L14 (128.6, -1.4) -> (1.4, -1.4)
  line L15 (1.4, -1.4) -> (1.4, -78.6)
  dimension "d246" = 0.6
extrude "Extrude55" add sketch "Sketch33" against normal blind 10 contours L0 L1 L2 L3 L8 L9 L10 L11 bodies 4
extrude "Extrude39" cut sketch "Sketch33" against normal blind 10 contours L12 L13 L14 L15 bodies 4
sketch "Sketch34" plane through (0, 0, 100) normal (0, 0, -1) x (1, 0, 0)
  line L0 (128.6, -78.6) -> (1.4, -78.6)
  line L1 (1.4, -78.6) -> (1.4, -1.4)
  line L2 (1.4, -1.4) -> (128.6, -1.4)
  line L3 (128.6, -1.4) -> (128.6, -78.6)
  line L4 (-25, -105) -> (155, -105)
  line L5 (155, -105) -> (155, 25)
  line L6 (155, 25) -> (-25, 25)
  line L7 (-25, 25) -> (-25, -105)
extrude "Extrude40" add sketch "Sketch34" against normal blind 5 contours L0 L1 L2 L3 bodies 4
sketch "Sketch35" plane through (0, 0, 75) normal (0, 0, 1) x (-1, 0, 0)
  line L0 (-2, -2) -> (-2, -78)
  line L1 (-2, -78) -> (-128, -78)
  line L2 (-128, -78) -> (-128, -2)
  line L3 (-128, -2) -> (-2, -2)
  line L4 (-130, -80) -> (0, -80)
  line L5 (0, -80) -> (0, 0)
  line L6 (0, 0) -> (-130, 0)
  line L7 (-130, 0) -> (-130, -80)
  line L8 (-2, -78) -> (-9, -78)
  line L9 (-9, -78) -> (-9, -2)
  line L10 (-128, -78) -> (-121, -78)
  line L11 (-121, -78) -> (-121, 0)
  line L12 (-128, -78) -> (-128, -71)
  line L13 (-128, -71) -> (-2, -71)
  line L14 (-2, -2) -> (-2, -9)
  line L15 (-2, -9) -> (-128, -9)
  line L16 (-20.0282, -2) -> (-20.0282, -9)
  line L17 (-76.1007, -2) -> (-76.1007, -9)
  dimension "d417" = 7
  dimension "d418" = 7
  dimension "d419" = 7
  dimension "d420" = 7
  constraint coincident L0.end L1.start
  constraint coincident L1 L8.end
  constraint coincident L3 L9.end
  constraint perpendicular L3 L9
  constraint coincident L1.end L2.start
  constraint coincident L1 L10.end
  constraint perpendicular L2 L10
  constraint coincident L6 L11.end
  constraint perpendicular L6 L11
  constraint coincident L2 L12.end
  constraint perpendicular L1 L12
  constraint coincident L0 L13.end
  constraint perpendicular L0 L13
  constraint coincident L0.start L3.end
  constraint coincident L0 L14.end
  constraint perpendicular L3 L14
  constraint coincident L2 L15.end
  constraint perpendicular L2 L15
  constraint coincident L3 L16.start
  constraint coincident L15 L16.end
  constraint perpendicular L15 L16
  constraint coincident L3 L17.start
  constraint coincident L15 L17.end
  constraint perpendicular L15 L17
  measures "d417" distance of L3 L15
  measures "d418" distance of L1 L13
  measures "d419" distance of L0 L9
  measures "d420" distance of L11 L12
extrude "Extrude41" add sketch "Sketch35" against normal blind 7 contours L0 L3 L9 L14 L15 | L0 L1 L8 L9 L13 | L1 L2 L10 L11 L12 L13 | L2 L3 L11 L15 bodies 1 2
sketch "Sketch36" plane through (0, 0, 75) normal (0, 0, 1) x (-1, 0, 0)
  line L0 (-2, -9) -> (-2, -71)
  line L1 (-9, -71) -> (-9, -78)
  line L2 (-9, -78) -> (-121, -78)
  line L3 (-121, -78) -> (-121, -71)
  line L4 (-128, -71) -> (-128, -9)
  line L5 (-121, -2) -> (-9, -2)
  line L6 (-130, -80) -> (0, -80)
  line L7 (0, -80) -> (0, 0)
  line L8 (0, 0) -> (-130, 0)
  line L9 (-130, 0) -> (-130, -80)
  circle A0 centre (-3.8154, -76.5304) radius 1.5
  circle A1 centre (-126.1011, -76.2995) radius 1.5
  circle A2 centre (-125.9478, -4.1031) radius 1.5
  circle A3 centre (-3.7387, -3.9492) radius 1.5
  line L10 (-2, -71) -> (-9, -71)
  line L11 (-121, -71) -> (-128, -71)
  line L12 (-128, -9) -> (-121, -9)
  line L13 (-121, -9) -> (-121, -2)
  line L14 (-9, -2) -> (-9, -9)
  line L15 (-9, -9) -> (-2, -9)
  dimension "d254" = 3
  dimension "d255" = 3
  dimension "d256" = 3
  dimension "d257" = 3
  measures "d254" diameter of A0
  measures "d255" diameter of A1
  measures "d256" diameter of A2
  measures "d257" diameter of A3
move_body "Move4" bodies 4 to x (1, 0, 0) y (0, 1, 0) z (0, 0, 1) at (0, 0, -25)
extrude "Extrude42" cut sketch "Sketch36" along normal blind 20 and the other way blind 7 contours A0 | A1 | A2 | A3 bodies 1 4